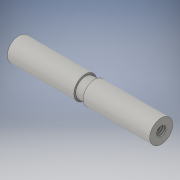
# Autodesk Inventor part: clawholder
Saved by Autodesk Inventor 2016 (Build 200138000, 138)
## iProperties
Created: 2015-05-24
Part Number: clawholder
Material: Generic
Document SubType Name: Modeling
Designer: Admin
Density: 1 g/cm^3
Appearance: Default
Author: Admin
Autodesk Inventor part; units mm, degrees
ref_plane "YZ Plane" through (0, 0, 0) normal (1, 0, 0) x (0, 1, 0)
ref_plane "XZ Plane" through (0, 0, 0) normal (0, 1, 0) x (-1, 0, 0)
ref_plane "XY Plane" through (0, 0, 0) normal (0, 0, 1) x (1, 0, 0)
sketch "Sketch1" plane through (0, 0, 0) normal (1, 0, 0) x (0, 1, 0)
  circle A0 centre (0, 0) radius 3.175
  dimension "d0" = 6.35
  constraints: 1 centre point, 1 coincident
  measures "d0" diameter of A0
extrude "Extrusion1" add sketch "Sketch1" along normal blind 39.37
sketch "Sketch2" plane through (39.37, 0, 0) normal (1, 0, 0) x (0, 0, -1)
  circle A0 centre (0, 0) radius 1.27
  dimension "d3" = 2.54
  constraints: 1 centre point, 1 coincident
  measures "d3" diameter of A0
extrude "Extrusion2" cut sketch "Sketch2" against normal blind 39.37
thread "Thread1" size "4-40 UNC" class "2B" standard "ANSI Unified Screw Threads" full length
sketch "Sketch5" plane through (0, 0, 0) normal (0, 1, 0) x (-1, 0, 0)
  line L0 (0, 0) -> (-39.37, 0)
  line L1 (-39.37, 3.175) -> (-39.37, -3.175) projected
  line L2 (0, -3.175) -> (-39.37, -3.175) projected
  line L3 (-19.685, -3.175) -> (-18.415, -3.175)
  line L4 (-18.415, -3.175) -> (-18.415, -2.667)
  line L5 (-18.415, -2.667) -> (-20.955, -2.667)
  line L6 (-20.955, -2.667) -> (-20.955, -3.175)
  line L7 (-20.955, -3.175) -> (-19.685, -3.175)
  dimension "d11" = 1.27
  dimension "d12" = 0.508
  dimension "d13" = 2.54
  constraints: 12 end point, 3 perpendicular, 2 midpoint, 2 point on line, 1 collinear
  measures "d11" distance of L3.start L3.end
  measures "d12" distance of L3.end L4.end
  measures "d13" distance of L4.end L5.end
revolve "Revolution1" cut sketch "Sketch5" angle 360 about axis through (0, 0, 0) along (1, 0, 0)
body "Solid1"
